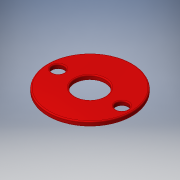
# Autodesk Inventor part: Steele Sewing Machine Bobbin Top
Saved by Autodesk Inventor 2016 (Build 200138000, 138)
## iProperties
Created: 2015-07-04
Part Number: Steele Sewing Machine Bobbin Top
Material: ABS Plastic
Document SubType Name: Modeling
Designer: steele
Density: 1.06 g/cm^3
Appearance: Red
Author: steele
Autodesk Inventor part; units mm, degrees
ref_plane "YZ Plane" through (0, 0, 0) normal (1, 0, 0) x (0, 1, 0)
ref_plane "XZ Plane" through (0, 0, 0) normal (0, 1, 0) x (-1, 0, 0)
ref_plane "XY Plane" through (0, 0, 0) normal (0, 0, 1) x (1, 0, 0)
sketch "Sketch1" plane through (0, 0, 0) normal (0, 1, 0) x (-1, 0, 0)
  circle A0 centre (0, 0) radius 10.2616
  circle A1 centre (0, 0) radius 3.6703
  dimension "d0" = 20.5232
  dimension "d1" = 7.3406
  constraints: 2 centre point, 2 coincident
  measures "d0" diameter of A0
  measures "d1" diameter of A1
extrude "Extrusion1" add sketch "Sketch1" along normal blind 1.143
sketch "Sketch3" plane through (0, 0, 0) normal (0, -1, 0) x (1, 0, 0)
  circle A0 centre (0, 0) radius 10.2616 construction
  line L0 (-10.2616, 0) -> (10.2616, 0) construction
  circle A1 centre (-7.7851, 0) radius 1.4478
  circle A2 centre (7.7851, 0) radius 1.4478
  dimension "d7" = 7.7851
  dimension "d8" = 2.8956
  dimension "d11" = 360
  constraints: 2 centre point, 2 end point, 2 point on circle, 1 horizontal, 1 point on line, 5 other
  measures "d7" distance of point (0, 0) A1.centre
  measures "d8" diameter of A1
extrude "Extrusion3" cut sketch "Sketch3" against normal through all
fillet "Fillet2" radius 0.254 8 edges at (10.2616, 1.143, 0) (6.3373, 1.143, 0) (3.6703, 1.143, 0) (-9.2329, 1.143, 0) (10.2616, 0, 0) (-9.2329, 0, 0) (6.3373, 0, 0) (3.6703, 0, 0)
body "Solid1"
